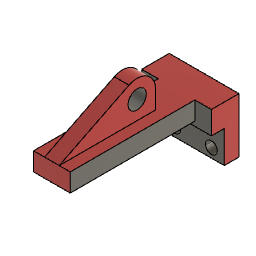
Figure-3 (Autodesk Fusion 360 design; units mm, degrees)
Autodesk Fusion 360 part; units mm, degrees
sketch "Sketch1" plane through (0, 0, 0) normal (0, 0, 1) x (1, 0, 0)
  line L0 (38, 8) -> (-38, 8)
  line L1 (-38, 8) -> (-38, -8)
  line L2 (-38, -8) -> (38, -8)
  line L3 (38, -8) -> (38, 8)
  line L4 (38, 8) -> (-38, -8) construction
  line L5 (-38, 8) -> (38, -8) construction
  dimension "d1" = 76
  dimension "d2" = 16
  constraint horizontal L0
  constraint perpendicular L0 L1
  constraint parallel L0 L2
  constraint parallel L1 L3
  constraint coincident L4 origin
  constraint coincident L5 origin
  measures "d1" distance of L1.end L2.end
  measures "d2" distance of L0.end L1.end
extrude "Extrude1" add sketch "Sketch1" along normal blind 60
sketch "Sketch2" plane through (0, 0, 60) normal (0, 0, 1) x (-1, 0, 0)
  line L0 (-38, 8) -> (-38, -8)
  line L1 (-38, -8) -> (38, -8)
  line L2 (38, -8) -> (38, 8)
  line L3 (38, 8) -> (-38, 8)
  line L4 (-38, -8) -> (-20, -8)
  line L5 (-20, -8) -> (-20, 22)
  line L6 (-20, 22) -> (-38, 22)
  line L7 (-38, 22) -> (-38, -8)
  line L8 (38, -8) -> (20, -8)
  line L9 (20, -8) -> (20, 22)
  line L10 (20, 22) -> (38, 22)
  line L11 (38, 22) -> (38, -8)
  dimension "d5" = 18
  dimension "d6" = 30
  dimension "d7" = 18
  dimension "d8" = 30
  constraint horizontal L4
  constraint vertical L5
  constraint horizontal L6
  constraint vertical L7
  constraint coincident L0.end L1.start
  constraint horizontal L8
  constraint vertical L9
  constraint horizontal L10
  constraint vertical L11
  constraint coincident L1.end L2.start
  measures "d5" distance of L0.end L4.end
  measures "d6" distance of L0.end L6.end
  measures "d7" distance of L1.end L8.end
  measures "d8" distance of L1.end L10.end
extrude "Extrude2" add sketch "Sketch2" against normal blind 25 contours L3 L5 L6 L7
extrude "Extrude3" add sketch "Sketch2" against normal blind 25 contours L3 L9 L10 L11
sketch "Sketch5" plane through (0, 0, 60) normal (0, 0, 1) x (-1, 0, 0)
  line L0 (-38, 22) -> (-38, -8)
  line L1 (-38, -8) -> (38, -8)
  line L2 (38, -8) -> (38, 22)
  line L3 (38, 22) -> (20, 22)
  line L4 (20, 22) -> (20, 8)
  line L5 (20, 8) -> (-20, 8)
  line L6 (-20, 8) -> (-20, 22)
  line L7 (-20, 22) -> (-38, 22)
  line L8 (20, 8) -> (-20, 8)
  line L9 (-20, 8) -> (-20, 158)
  line L10 (-20, 158) -> (20, 158)
  line L11 (20, 158) -> (20, 8)
  dimension "d18" = 40
  dimension "d19" = 150
  constraint horizontal L8
  constraint vertical L9
  constraint horizontal L10
  constraint vertical L11
  constraint coincident L4.end L5.start
  measures "d18" distance of L4.end L5.end
  measures "d19" distance of L4.end L10.end
extrude "Extrude5" add sketch "Sketch5" against normal blind 20 contours L4 L5 L6 L8 L9 L10 L11
sketch "Sketch6" plane through (0, 0, 60) normal (0, 0, 1) x (-1, 0, 0)
  line L0 (-38, 22) -> (-38, -8)
  line L1 (-38, -8) -> (38, -8)
  line L2 (38, -8) -> (38, 22)
  line L3 (38, 22) -> (20, 22)
  line L4 (20, 22) -> (20, 158)
  line L5 (20, 158) -> (-20, 158)
  line L6 (-20, 158) -> (-20, 22)
  line L7 (-20, 22) -> (-38, 22)
  line L8 (-20, 22, -25) -> (20, 22, -25)
  line L9 (20, 22, -25) -> (20, 8, -25)
  line L10 (20, 8, -25) -> (-20, 8, -25)
  line L11 (-20, 8, -25) -> (-20, 22, -25)
  point P0 (-20, 22)
  point P1 (20, 8)
  constraint coincident P0 L6.end
extrude "Extrude6" add sketch "Sketch6" along normal blind 15 contours L8 L9 L10 L11 in plane through (0, 0, 35) normal (0, 0, 1)
sketch "Sketch7" plane through (0, -8, 0) normal (0, -1, 0) x (1, 0, 0)
  line L0 (38, 35) -> (-38, 35)
  line L1 (-38, 35) -> (-38, 0)
  line L2 (-38, 0) -> (38, 0)
  line L3 (38, 0) -> (38, 35)
  circle A0 centre (24, 10) radius 6.5
  circle A1 centre (-16, 10) radius 6.5
  point P0 (38, 0)
  point P1 (24, 0)
  point P2 (-16, 0)
  point P3 (38, 10)
  dimension "d24" = 14
  dimension "d25" = 40
  dimension "d26" = 10
  dimension "d27" = 13
  dimension "d28" = 13
  constraint coincident P0 L2.end
  constraint coincident L2 P1
  constraint coincident L2 P2
  constraint coincident L3 P3
  measures "d24" distance of P0 P1
  measures "d25" distance of P1 P2
  measures "d26" distance of P0 P3
  measures "d27" diameter of A0
  measures "d28" diameter of A1
extrude "Extrude7" cut sketch "Sketch7" against normal blind 280 contours A1
extrude "Extrude8" cut sketch "Sketch7" against normal blind 190 contours A0
sketch "Sketch14" plane through (0, -105.5, 75) normal (-1, 0, 0) x (0, 0, -1)
  line L0 (15, 52.5) -> (-22.9016, -23.582)
  line L1 (15, 52.5) -> (15, -52.5)
  line L2 (15, -52.5) -> (-25, -52.5)
  line L3 (-25, -52.5) -> (-25, -32.5)
  arc A0 (-22.9016, -23.582) -> (-25, -32.5) centre (-5, -32.5) ccw
  point P0 (-5, -32.5)
  point P1 (15, 52.5)
  point P2 (15, -52.5)
  dimension "d56" = 40
  constraint coincident P0 A0.centre
  constraint coincident P1 L0.start
  constraint tangent L0 A0
  constraint coincident P2 L1.end
  constraint perpendicular L1 L2
  constraint tangent L3 A0
  constraint perpendicular L2 L3
  measures "d56" diameter of A0
sketch "Sketch15" plane through (0, -105.5, 75) normal (-1, 0, 0) x (0, 0, -1)
  circle A0 centre (-5, -32.5) radius 10
  point P0 (-5, -32.5)
  dimension "d57" = 20
  constraint coincident P0 A0.centre
  measures "d57" diameter of A0
extrude "Extrude10" add sketch "Sketch14" along normal mid plane 16
extrude "Extrude11" cut sketch "Sketch15" along normal through all and the other way through all
fillet "Fillet1" radius 20 1 edges at (0, -53, 100)
extrude "Extrude4" [rolled back] along distance -20 taper angle 0
sketch "Sketch4" plane through (0, 0, 60) normal (0, 0, 1) x (-1, 0, 0)
  line L0 (-38, 22) -> (-38, -8)
  line L1 (-38, -8) -> (38, -8)
  line L2 (38, -8) -> (38, 22)
  line L3 (38, 22) -> (20, 22)
  line L4 (20, 22) -> (20, 142)
  line L5 (20, 142) -> (-20, 142)
  line L6 (-20, 142) -> (-20, 22)
  line L7 (-20, 22) -> (-38, 22)
  line L8 (0, 142, 0) -> (17.0332, 39.8005, -17.0332)
  point P0 (0, 142)
  dimension "d17" = 105
